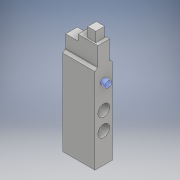
# Autodesk Inventor part: solenoid _valve_sa
Saved by Autodesk Inventor 2018 (Build 220112000, 112)
## iProperties
Created: 2018-03-07
Part Number: solenoid _valve_sa
Material: 一般
Document SubType Name: Modeling
Designer: shun
Density: 1 g/cm^3
Appearance: 既定
Author: shun
Autodesk Inventor part; units mm, degrees
ref_plane "YZ Plane" through (0, 0, 0) normal (1, 0, 0) x (0, 1, 0)
ref_plane "XZ Plane" through (0, 0, 0) normal (0, 1, 0) x (-1, 0, 0)
ref_plane "XY Plane" through (0, 0, 0) normal (0, 0, 1) x (1, 0, 0)
sketch "スケッチ1" plane through (0, 0, 0) normal (0, 0, 1) x (1, 0, 0)
  line L0 (-13.75, -7.5) -> (13.75, -7.5)
  line L1 (13.75, -7.5) -> (13.75, 7.5)
  line L2 (13.75, 7.5) -> (-13.75, 7.5)
  line L3 (-13.75, 7.5) -> (-13.75, -7.5)
  line L4 (-13.75, -7.5) -> (13.75, 7.5) construction
  line L5 (13.75, -7.5) -> (-13.75, 7.5) construction
  point P0 (0, 0)
  dimension "d0" = 27.5
  dimension "d1" = 15
  constraints: 12 end point, 2 midpoint, 2 parallel, 1 horizontal, 1 perpendicular
  measures "d0" distance of L2.end L1.end
  measures "d1" distance of L1.end L0.end
extrude "押し出し1" add sketch "スケッチ1" along normal blind 75
sketch "スケッチ2" plane through (0, 0, 75) normal (0, 0, 1) x (1, 0, 0)
  line L0 (-13.75, 5) -> (13.75, 5)
  line L1 (13.75, 5) -> (13.75, -5)
  line L2 (13.75, -5) -> (-13.75, -5)
  line L3 (-13.75, -5) -> (-13.75, 5)
  line L4 (-13.75, 5) -> (13.75, -5) construction
  line L5 (13.75, 5) -> (-13.75, -5) construction
  point P0 (0, 0)
  dimension "d4" = 27.5
  dimension "d5" = 10
  constraints: 12 end point, 2 midpoint, 2 parallel, 1 horizontal, 1 perpendicular
  measures "d4" distance of L1.end L2.end
  measures "d5" distance of L0.end L1.end
extrude "押し出し2" add sketch "スケッチ2" along normal blind 11
chamfer "面取り1" distance 2 angle 45 2 edges at (0, 7.5, 75) (0, -7.5, 75)
sketch "スケッチ3" plane through (0, 0, 86) normal (0, 0, 1) x (1, 0, 0)
  line L0 (13.75, -5) -> (13.75, 5) projected
  line L1 (13.75, -5) -> (-13.75, -5) projected
  line L2 (13.75, 5) -> (-3.25, 5)
  line L3 (-3.25, 5) -> (-3.25, -5)
  line L4 (-3.25, -5) -> (13.75, -5)
  line L5 (13.75, -5) -> (13.75, 5)
  point P0 (0, 0)
  dimension "d11" = 17
  constraints: 8 end point, 2 parallel, 1 horizontal, 1 perpendicular, 1 point on line
  measures "d11" distance of L4.end L3.end
extrude "押し出し3" add sketch "スケッチ3" along normal blind 5
sketch "スケッチ4" plane through (0, 0, 91) normal (0, 0, 1) x (1, 0, 0)
  line L0 (3.75, -3.75) -> (10.75, -3.75)
  line L1 (10.75, -3.75) -> (10.75, 3.75)
  line L2 (10.75, 3.75) -> (3.75, 3.75)
  line L3 (3.75, 3.75) -> (3.75, -3.75)
  line L4 (3.75, -3.75) -> (10.75, 3.75) construction
  line L5 (10.75, -3.75) -> (3.75, 3.75) construction
  line L6 (13.75, -5) -> (13.75, 5) projected
  point P0 (0, 0)
  point P1 (7.25, 0)
  dimension "d14" = 7
  dimension "d15" = 7.5
  dimension "d16" = 3
  constraints: 12 end point, 2 midpoint, 2 parallel, 1 horizontal, 1 perpendicular
  measures "d14" distance of L2.end L1.end
  measures "d15" distance of L1.end L0.end
  measures "d16" distance between parallel lines of L6 L1
extrude "押し出し4" add sketch "スケッチ4" along normal blind 8.5
sketch "スケッチ5" plane through (13.75, -7.5, 0) normal (1, 0, 0) x (0, 0, -1)
  line L0 (0, 7.5) -> (-91, 7.5) construction
  line L1 (-91, 2.5) -> (-91, 12.5) projected
  line L2 (0, 0) -> (0, 15) projected
  point P0 (-25.5, 7.5)
  point P1 (-40.5, 7.5)
  dimension "d19" = 25.5
  dimension "d20" = 15
  constraints: 2 end point, 2 point on line, 1 midpoint
  measures "d19" distance from line of L2 point (-25.5, 7.5)
  measures "d20" distance of point (-25.5, 7.5) point (-40.5, 7.5)
hole "穴1" at (13.75, 0, 25.5) at (13.75, 0, 40.5) direction (-1, 0, 0) diameter 10 depth 8 tip angle 118
sketch "スケッチ6" plane through (-13.75, -7.5, 0) normal (-1, 0, 0) x (0, 0, 1)
  line L0 (0, 7.5) -> (86, 7.5) construction
  line L1 (86, 2.5) -> (86, 12.5) projected
  line L2 (0, 15) -> (0, 0) projected
  point P0 (34, 7.5)
  point P1 (19, 7.5)
  point P2 (49, 7.5)
  dimension "d28" = 19
  dimension "d29" = 15
  dimension "d30" = 15
  constraints: 3 point on line, 2 end point, 1 midpoint
  measures "d28" distance from line of L2 point (19, 7.5)
  measures "d29" distance of point (34, 7.5) point (19, 7.5)
  measures "d30" distance of point (49, 7.5) point (34, 7.5)
hole "穴2" at (-13.75, 0, 34) at (-13.75, 0, 19) at (-13.75, 0, 49) direction (1, 0, 0) diameter 10 depth 8 tip angle 118
sketch "スケッチ7" plane through (-13.75, 7.5, 0) normal (0, 1, 0) x (1, 0, 0)
  line L0 (27.5, 0) -> (0, 0) projected
  line L1 (5, 0) -> (5, -72.92) construction
  line L2 (0, 0) -> (0, -73) projected
  point P0 (13.75, 0)
  point P1 (5, -26)
  point P2 (5, -39.5)
  dimension "d38" = 5
  dimension "d39" = 26
  dimension "d40" = 13.5
  constraints: 3 point on line, 2 end point, 1 vertical
  measures "d38" distance between parallel lines of L1 L2
  measures "d39" distance from line of L0 point (5, -26)
  measures "d40" distance of point (5, -39.5) point (5, -26)
hole "穴3" at (-8.75, 7.5, 26) at (-8.75, 7.5, 39.5) direction (0, -1, 0) diameter 3 depth 8 tip angle 118
sketch "スケッチ8" plane through (13.75, -7.5, 0) normal (1, 0, 0) x (0, 0, -1)
  line L0 (0, 7.5) -> (-99.5, 7.5) construction
  line L1 (-99.5, 3.75) -> (-99.5, 11.25) projected
  circle A0 centre (-62, 7.5) radius 2.75
  line L2 (0, 0) -> (0, 15) projected
  dimension "d48" = 5.5
  dimension "d49" = 62
  constraints: 2 end point, 1 centre point, 1 midpoint, 1 point on line
  measures "d48" diameter of A0
  measures "d49" distance from line of L2 A0.centre
extrude "押し出し5" add sketch "スケッチ8" along normal blind 4
